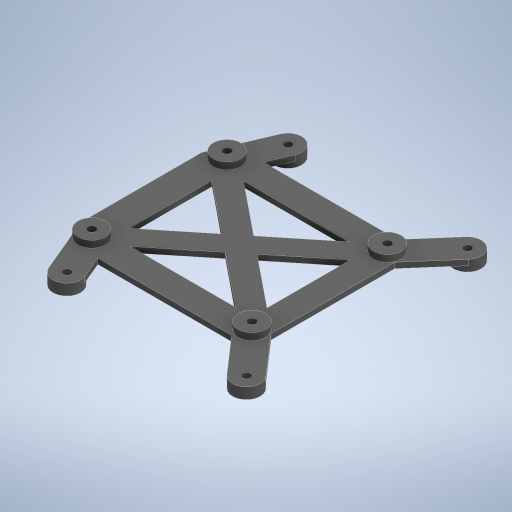
# Autodesk Inventor part: board_connector
Saved by Autodesk Inventor 2024.1 (Build 281209000, 209)
## iProperties
Created: 2024-08-02
Part Number: board_connector
Material: 一般
Document SubType Name: Modeling
Designer: hibik
Density: 1 g/cm^3
Appearance: 既定
Author: hibik
Autodesk Inventor part; units mm, degrees
ref_plane "YZ Plane" through (0, 0, 0) normal (1, 0, 0) x (0, 1, 0)
ref_plane "XZ Plane" through (0, 0, 0) normal (0, 1, 0) x (-1, 0, 0)
ref_plane "XY Plane" through (0, 0, 0) normal (0, 0, 1) x (1, 0, 0)
sketch "スケッチ1" plane through (0, 0, 0) normal (0, 1, 0) x (-1, 0, 0)
  line L0 (37.5, 45) -> (-37.5, 45) construction
  line L1 (-37.5, 45) -> (-37.5, -45) construction
  line L2 (-37.5, -45) -> (37.5, -45) construction
  line L3 (37.5, -45) -> (37.5, 45) construction
  circle A0 centre (32.5, 40) radius 1.5
  circle A1 centre (32.5, -40) radius 1.5
  circle A2 centre (-32.5, -40) radius 1.5
  circle A3 centre (-32.5, 40) radius 1.5
  line L4 (39, 24.5) -> (-39, 24.5) construction
  line L5 (-39, 24.5) -> (-39, -24.5) construction
  line L6 (-39, -24.5) -> (39, -24.5) construction
  line L7 (39, -24.5) -> (39, 24.5) construction
  line L8 (39, 24.5) -> (-39, -24.5) construction
  line L9 (-39, 24.5) -> (39, -24.5) construction
  line L10 (-19, 24.5) -> (-19, -24.5) construction
  circle A4 centre (39, 24.5) radius 1.5
  circle A5 centre (39, -24.5) radius 1.5
  circle A6 centre (-19, -24.5) radius 1.5
  circle A7 centre (-19, 24.5) radius 1.5
  line L11 (-32.0135, -47.0543) -> (-39.5543, -40.4865)
  line L12 (-39.5543, -40.4865) -> (-19.4865, -17.4457)
  line L13 (-19.4865, -17.4457) -> (-11.9457, -24.0135)
  line L14 (-11.9457, -24.0135) -> (-32.0135, -47.0543)
  line L15 (32.5, 40) -> (39, 24.5)
  line L16 (39, -24.5) -> (32.5, -40)
  line L17 (-19, -24.5) -> (-32.5, -40)
  line L18 (-19, 24.5) -> (-32.5, 40)
  line L19 (45.5446, 21.8227) -> (36.3227, 17.9554)
  line L20 (36.3227, 17.9554) -> (25.9554, 42.6773)
  line L21 (25.9554, 42.6773) -> (35.1773, 46.5446)
  line L22 (35.1773, 46.5446) -> (45.5446, 21.8227)
  line L23 (45.5446, -21.8227) -> (36.3227, -17.9554)
  line L24 (36.3227, -17.9554) -> (25.9554, -42.6773)
  line L25 (25.9554, -42.6773) -> (35.1773, -46.5446)
  line L26 (35.1773, -46.5446) -> (45.5446, -21.8227)
  line L27 (-32.0135, 47.0543) -> (-39.5543, 40.4865)
  line L28 (-39.5543, 40.4865) -> (-19.4865, 17.4457)
  line L29 (-19.4865, 17.4457) -> (-11.9457, 24.0135)
  line L30 (-11.9457, 24.0135) -> (-32.0135, 47.0543)
  line L31 (45.5446, 30) -> (-23.7903, 30)
  line L32 (-23.7903, 30) -> (-23.7903, -30)
  line L33 (-23.7903, -30) -> (45.5446, -30)
  line L34 (45.5446, -30) -> (45.5446, 30)
  point P0 (0, 0)
  point P1 (40.9336, 19.889)
  point P2 (-15.7161, -20.7296)
  point P3 (40.9336, -19.889)
  point P4 (-15.7161, 20.7296)
  point P5 (-17.1597, -30)
  point P6 (31.2717, -30)
  point P7 (45.5446, -21.8227)
  point P8 (31.2717, 30)
  point P9 (-17.1597, 30)
  point P10 (-23.7903, 22.3871)
  point P11 (-23.7903, -22.3871)
  point P12 (37.5, 0)
  point P13 (0, -45)
  dimension "d0" = 75
  dimension "d1" = 90
  dimension "d2" = 3
  dimension "d3" = 5
  dimension "d4" = 78
  dimension "d5" = 49
  dimension "d6" = 58
  dimension "d8" = 10
  dimension "d9" = 5
  dimension "d10" = 5
  dimension "d11" = 5
  dimension "d12" = 5
  dimension "d13" = 5
  dimension "d14" = 5
  dimension "d15" = 5
  dimension "d16" = 5
  dimension "d17" = 60
  dimension "d48" = 5
  dimension "d49" = 5
  dimension "d50" = 5
  constraints: 70 end point, 18 parallel, 9 point on line, 8 centre point, 8 midpoint, 8 perpendicular, 7 equal radius, 4 coincident, 3 equal length, 3 horizontal, 3 horizontal alignment, 3 vertical alignment
  measures "d0" distance of L2.end L1.end
  measures "d1" distance of L1.end L0.end
  measures "d2" diameter of A0
  measures "d3" distance from line of L3 L15.start
  measures "d4" distance of L6.end L5.end
  measures "d5" distance of L5.end L4.end
  measures "d6" distance between parallel lines of L7 L10
  measures "d8" distance between parallel lines of L22 L20
  measures "d9" distance from line of L19 L4.start
  measures "d10" distance from line of L15.start L21
  measures "d11" distance from line of L23 L6.end
  measures "d12" distance from line of L25 L16.end
  measures "d13" distance from line of L29 L10.start
  measures "d14" distance from line of L27 L18.end
  measures "d15" distance from line of L13 L17.start
  measures "d16" distance from line of L11 L17.end
  measures "d17" distance of L33.end L31.start
  measures "d48" distance from line of L0 L15.start
  measures "d49" distance from line of L2 L16.end
  measures "d50" distance from line of L1 L18.end
extrude "押し出し1" add sketch "スケッチ1" along normal blind 2 contours L11 L12 L32 L33 L14 | L33 L32 L12 L13 L14 | L14 L13 L12 L32 L28 L29 L30 L31 L20 L19 L34 L23 L24 L33 | L33 L26 L25 L24 | L24 L23 L26 L33 | L32 L31 L30 L29 L28 | L28 L27 L30 L31 L32 | L19 L20 L31 L22 | L20 L21 L22 L31
sketch "スケッチ2" plane through (0, 2, 0) normal (0, 1, 0) x (1, 0, 0)
  circle A0 centre (-39, 24.5) radius 1.5 projected
  circle A1 centre (19, -24.5) radius 1.5 projected
  line L0 (-39, 24.5) -> (19, 24.5) construction
  line L1 (19, 24.5) -> (19, -24.5) construction
  line L2 (19, -24.5) -> (-39, -24.5) construction
  line L3 (-39, -24.5) -> (-39, 24.5) construction
  line L4 (-35, 20.5) -> (15, 20.5)
  line L5 (15, 20.5) -> (15, -20.5)
  line L6 (15, -20.5) -> (-35, -20.5)
  line L7 (-35, -20.5) -> (-35, 20.5)
  line L8 (-33.9741, 24.5) -> (19, -18.2758)
  line L9 (19, -18.2758) -> (13.9741, -24.5)
  line L10 (13.9741, -24.5) -> (-39, 18.2758)
  line L11 (-39, 18.2758) -> (-33.9741, 24.5)
  line L12 (-33.9741, 24.5) -> (13.9741, -24.5) construction
  line L13 (19, -18.2758) -> (-39, 18.2758) construction
  line L14 (-39, -18.2758) -> (13.9741, 24.5)
  line L15 (13.9741, 24.5) -> (19, 18.2758)
  line L16 (19, 18.2758) -> (-33.9741, -24.5)
  line L17 (-33.9741, -24.5) -> (-39, -18.2758)
  line L18 (-39, -18.2758) -> (19, 18.2758) construction
  line L19 (13.9741, 24.5) -> (-33.9741, -24.5) construction
  point P0 (0, 0)
  point P1 (-10, 0)
  point P2 (-10, 0)
  point P3 (-10, -5.1413)
  point P4 (-29.0204, -20.5)
  point P5 (9.0204, -20.5)
  point P6 (15, 15.0459)
  point P7 (-3.633, 0)
  point P8 (15, -15.0459)
  point P9 (-10, 5.1413)
  point P10 (9.0204, 20.5)
  point P11 (-29.0204, 20.5)
  point P12 (-35, -15.0459)
  point P13 (-16.367, 0)
  point P14 (-35, 15.0459)
  dimension "d20" = 4
  dimension "d21" = 4
  dimension "d22" = 4
  dimension "d23" = 4
  dimension "d24" = 8
  constraints: 40 end point, 8 parallel, 6 point on line, 5 midpoint, 4 perpendicular, 2 horizontal, 1 equal length
  measures "d20" distance between parallel lines of L3 L7
  measures "d21" distance between parallel lines of L0 L4
  measures "d22" distance between parallel lines of L1 L5
  measures "d23" distance between parallel lines of L2 L6
  measures "d24" distance between parallel lines of L16 L14
extrude "押し出し2" cut sketch "スケッチ2" against normal through all contours L4 L14 L8 | L10 L14 L7 | L16 L5 L8 | L10 L6 L16
sketch "スケッチ3" plane through (0, 2, 0) normal (0, 1, 0) x (1, 0, 0)
  circle A0 centre (-39, 24.5) radius 1.5 projected
  circle A1 centre (19, 24.5) radius 1.5 projected
  circle A2 centre (19, -24.5) radius 1.5 projected
  circle A3 centre (-39, -24.5) radius 1.5 projected
  circle A4 centre (-39, 24.5) radius 5
  circle A5 centre (19, 24.5) radius 5
  circle A6 centre (19, -24.5) radius 5
  circle A7 centre (-39, -24.5) radius 5
  point P0 (0, 0)
  dimension "d27" = 10
  constraints: 4 centre point, 4 coincident, 3 equal radius
  measures "d27" diameter of A4
extrude "押し出し3" add sketch "スケッチ3" along normal blind 2.5
sketch "スケッチ4" plane through (0, 0, 0) normal (0, -1, 0) x (1, 0, 0)
  line L0 (-41.3094, 20.5) -> (-43.6188, 24.5)
  line L1 (-43.6188, 24.5) -> (-41.3094, 28.5)
  line L2 (-41.3094, 28.5) -> (-36.6906, 28.5)
  line L3 (-36.6906, 28.5) -> (-34.3812, 24.5)
  line L4 (-34.3812, 24.5) -> (-36.6906, 20.5)
  line L5 (-36.6906, 20.5) -> (-41.3094, 20.5)
  line L6 (16.6906, 20.5) -> (14.3812, 24.5)
  line L7 (14.3812, 24.5) -> (16.6906, 28.5)
  line L8 (16.6906, 28.5) -> (21.3094, 28.5)
  line L9 (21.3094, 28.5) -> (23.6188, 24.5)
  line L10 (23.6188, 24.5) -> (21.3094, 20.5)
  line L11 (21.3094, 20.5) -> (16.6906, 20.5)
  circle A0 centre (19, -24.5) radius 1.5 projected
  line L12 (16.6906, -20.5) -> (21.3094, -20.5)
  line L13 (21.3094, -20.5) -> (23.6188, -24.5)
  line L14 (23.6188, -24.5) -> (21.3094, -28.5)
  line L15 (21.3094, -28.5) -> (16.6906, -28.5)
  line L16 (16.6906, -28.5) -> (14.3812, -24.5)
  line L17 (14.3812, -24.5) -> (16.6906, -20.5)
  circle A1 centre (-39, -24.5) radius 1.5 projected
  line L18 (-36.6906, -20.5) -> (-34.3812, -24.5)
  line L19 (-34.3812, -24.5) -> (-36.6906, -28.5)
  line L20 (-36.6906, -28.5) -> (-41.3094, -28.5)
  line L21 (-41.3094, -28.5) -> (-43.6188, -24.5)
  line L22 (-43.6188, -24.5) -> (-41.3094, -20.5)
  line L23 (-41.3094, -20.5) -> (-36.6906, -20.5)
  point P0 (-39, 24.5)
  point P1 (19, 24.5)
  point P2 (-39, 24.5)
  point P3 (19, 24.5)
  point P4 (19, 24.5)
  dimension "d32" = 8
  constraints: 48 end point, 4 coincident, 4 horizontal, 3 equal length, 51 other
  measures "d32" distance between parallel lines of L5 L2
extrude "押し出し4" cut sketch "スケッチ4" against normal blind 2 contours L0 L1 L2 L3 L4 L5 | L6 L7 L8 L9 L10 L11 | A0 | L12 L13 L14 L15 L16 L17 | A1 | L18 L19 L20 L21 L22 L23
sketch "スケッチ5" plane through (0, 0, 0) normal (0, -1, 0) x (1, 0, 0)
  circle A0 centre (-32.5, -40) radius 1.5 projected
  circle A1 centre (32.5, -40) radius 1.5 projected
  circle A2 centre (32.5, 40) radius 1.5 projected
  circle A3 centre (-32.5, 40) radius 1.5 projected
  circle A4 centre (-32.5, -40) radius 5
  circle A5 centre (-32.5, 40) radius 5
  circle A6 centre (32.5, 40) radius 5
  circle A7 centre (32.5, -40) radius 5
  point P0 (0, 0)
  dimension "d35" = 10
  constraints: 4 centre point, 4 coincident, 3 equal radius
  measures "d35" diameter of A4
extrude "押し出し5" add sketch "スケッチ5" along normal blind 2
fillet "フィレット1" radius 5 8 edges at (32.0135, 1, -47.0543) (39.5543, 1, -40.4865) (39.5543, 1, 40.4865) (32.0135, 1, 47.0543) (-35.1773, 1, 46.5446) (-25.9554, 1, 42.6773) (-25.9554, 1, -42.6773) (-35.1773, 1, -46.5446)
equation "\"d10\" = d9"
equation "\"d11\" = d9"
equation "\"d12\" = d11"
equation "\"d13\" = d9"
equation "\"d14\" = d10"
equation "\"d15\" = d9"
equation "\"d16\" = d15"
equation "\"d21\" = d20"
equation "\"d22\" = d20"
equation "\"d23\" = d20"
